Autodesk Fusion 360 part; units mm, degrees
(part 3 of 4)
  spline S333 degree 3 poles (-231.1347, 101.123) (-229.8927, 98.7978) (-228.9901, 97.7435) (-226.7371, 95.9744) knots 0 0 0 0 1 1 1 1
  spline S334 degree 3 poles (-226.7371, 95.9744) (-226.2605, 95.6061) (-225.5529, 95.0284) (-225.1629, 94.6962) knots 0 0 0 0 1 1 1 1
  spline S335 degree 3 poles (-225.1629, 94.6962) (-224.383, 94.0175) (-224.3903, 94.0319) (-224.5708, 93.2665) knots 0 0 0 0 1 1 1 1
  spline S336 degree 3 poles (-224.5708, 93.2665) (-224.8163, 92.2483) (-224.6574, 91.194) (-224.1087, 90.1614) knots 0 0 0 0 1 1 1 1
  spline S337 degree 3 poles (-224.1087, 90.1614) (-223.762, 89.5115) (-223.7548, 89.4754) (-223.7332, 88.3417) knots 0 0 0 0 1 1 1 1
  line L62 (-223.7332, 88.3417) -> (-223.7115, 87.3886)
  line L63 (-223.7115, 87.3886) -> (-224.1231, 87.1719)
  spline S338 degree 3 poles (-224.1231, 87.1719) (-224.9607, 86.7314) (-225.9717, 85.8144) (-227.0765, 84.4929) knots 0 0 0 0 1 1 1 1
  spline S339 degree 3 poles (-227.0765, 84.4929) (-227.8564, 83.5686) (-228.8168, 82.11) (-229.1128, 81.4168) knots 0 0 0 0 1 1 1 1
  spline S340 degree 3 poles (-229.1128, 81.4168) (-229.2428, 81.099) (-229.5244, 80.4708) (-229.7266, 80.0159) knots 0 0 0 0 1 1 1 1
  spline S341 degree 3 poles (-229.7266, 80.0159) (-230.6942, 77.8857) (-231.1925, 75.6399) (-231.0264, 74.1668) knots 0 0 0 0 1 1 1 1
  spline S342 degree 3 poles (-231.0264, 74.1668) (-230.817, 72.3038) (-229.9071, 71.3073) (-228.1091, 70.9679) knots 0 0 0 0 1 1 1 1
  spline S343 degree 3 poles (-228.1091, 70.9679) (-226.441, 70.6502) (-226.4844, 70.6502) (-225.7839, 70.9318) knots 0 0 0 0 1 1 1 1
  spline S344 degree 3 poles (-225.7839, 70.9318) (-225.4445, 71.069) (-225.3796, 71.0762) (-225.1196, 70.9896) knots 0 0 0 0 1 1 1 1
  spline S345 degree 3 poles (-225.1196, 70.9896) (-224.8669, 70.9101) (-224.7513, 70.9101) (-224.282, 71.0257) knots 0 0 0 0 1 1 1 1
  spline S346 degree 3 poles (-224.282, 71.0257) (-223.6754, 71.1701) (-223.1266, 71.1412) (-222.6717, 70.9463) knots 0 0 0 0 1 1 1 1
  spline S347 degree 3 poles (-222.6717, 70.9463) (-222.5272, 70.8813) (-222.1806, 70.8018) (-221.9062, 70.7657) knots 0 0 0 0 1 1 1 1
  spline S348 degree 3 poles (-221.9062, 70.7657) (-221.6174, 70.7296) (-221.1986, 70.6069) (-220.9458, 70.4913) knots 0 0 0 0 1 1 1 1
  spline S349 degree 3 poles (-220.9458, 70.4913) (-220.4692, 70.2603) (-219.7977, 69.6826) (-219.545, 69.2854) knots 0 0 0 0 1 1 1 1
  spline S350 degree 3 poles (-219.545, 69.2854) (-219.3428, 68.9532) (-219.1839, 68.9244) (-218.729, 69.1338) knots 0 0 0 0 1 1 1 1
  spline S351 degree 3 poles (-218.729, 69.1338) (-217.3498, 69.762) (-215.9489, 71.069) (-214.3964, 73.1559) knots 0 0 0 0 1 1 1 1
  spline S352 degree 3 poles (-214.3964, 73.1559) (-213.8548, 73.8924) (-213.3782, 74.499) (-213.3421, 74.5134) knots 0 0 0 0 1 1 1 1
  spline S353 degree 3 poles (-213.3421, 74.5134) (-213.2338, 74.5496) (-206.4099, 71.1268) (-206.4099, 71.0329) knots 0 0 0 0 1 1 1 1
  spline S354 degree 3 poles (-206.4099, 71.0329) (-206.4099, 70.9896) (-206.4821, 70.8379) (-206.5688, 70.7007) knots 0 0 0 0 1 1 1 1
  spline S355 degree 3 poles (-206.5688, 70.7007) (-206.9731, 70.0364) (-207.2403, 69.5165) (-207.7747, 68.3322) knots 0 0 0 0 1 1 1 1
  spline S356 degree 3 poles (-207.7747, 68.3322) (-208.4318, 66.8664) (-208.5618, 66.462) (-208.6195, 65.7543) knots 0 0 0 0 1 1 1 1
  spline S357 degree 3 poles (-208.6195, 65.7543) (-208.6484, 65.3644) (-208.6268, 65.1622) (-208.5257, 64.8878) knots 0 0 0 0 1 1 1 1
  spline S358 degree 3 poles (-208.5257, 64.8878) (-208.4101, 64.5701) (-208.3596, 64.5268) (-208.1646, 64.5051) knots 0 0 0 0 1 1 1 1
  spline S359 degree 3 poles (-208.1646, 64.5051) (-207.8324, 64.469) (-207.6591, 64.2307) (-207.5364, 63.6458) knots 0 0 0 0 1 1 1 1
  spline S360 degree 3 poles (-207.5364, 63.6458) (-207.4064, 63.0031) (-207.2692, 62.7432) (-206.9731, 62.5265) knots 0 0 0 0 1 1 1 1
  spline S361 degree 3 poles (-206.9731, 62.5265) (-206.7421, 62.3677) (-206.6843, 62.3604) (-205.3267, 62.3604) knots 0 0 0 0 1 1 1 1
  spline S362 degree 3 poles (-205.3267, 62.3604) (-203.9692, 62.3604) (-203.9114, 62.3532) (-203.6803, 62.1944) knots 0 0 0 0 1 1 1 1
  spline S363 degree 3 poles (-203.6803, 62.1944) (-203.5504, 62.1005) (-203.3626, 61.8622) (-203.2687, 61.6672) knots 0 0 0 0 1 1 1 1
  spline S364 degree 3 poles (-203.2687, 61.6672) (-203.0377, 61.2195) (-202.8716, 61.1256) (-202.5033, 61.234) knots 0 0 0 0 1 1 1 1
  spline S365 degree 3 poles (-202.5033, 61.234) (-202.0773, 61.3639) (-201.5429, 61.9055) (-200.597, 63.1764) knots 0 0 0 0 1 1 1 1
  spline S366 degree 3 poles (-200.597, 63.1764) (-199.586, 64.5268) (-198.6617, 66.0937) (-198.2862, 67.0902) knots 0 0 0 0 1 1 1 1
  spline S367 degree 3 poles (-198.2862, 67.0902) (-197.9396, 68.0001) (-197.6724, 68.8016) (-197.6724, 68.9244) knots 0 0 0 0 1 1 1 1
  spline S368 degree 3 poles (-197.6724, 68.9244) (-197.6724, 69.1627) (-197.4847, 69.1915) (-197.0587, 69.0038) knots 0 0 0 0 1 1 1 1
  spline S369 degree 3 poles (-197.0587, 69.0038) (-196.5893, 68.7944) (-194.9285, 68.3467) (-193.4409, 68.029) knots 0 0 0 0 1 1 1 1
  spline S370 degree 3 poles (-193.4409, 68.029) (-192.1772, 67.7546) (-191.8956, 67.6029) (-191.7512, 67.1263) knots 0 0 0 0 1 1 1 1
  spline S371 degree 3 poles (-191.7512, 67.1263) (-191.6718, 66.8664) (-191.5346, 66.657) (-191.2168, 66.3392) knots 0 0 0 0 1 1 1 1
  line L64 (-191.2168, 66.3392) -> (-190.7908, 65.906)
  line L65 (-190.7908, 65.906) -> (-190.2059, 65.906)
  spline S372 degree 3 poles (-190.2059, 65.906) (-189.7149, 65.8988) (-189.5849, 65.8699) (-189.3899, 65.7327) knots 0 0 0 0 1 1 1 1
  spline S373 degree 3 poles (-189.3899, 65.7327) (-188.9567, 65.4222) (-188.8267, 65.1622) (-188.8267, 64.599) knots 0 0 0 0 1 1 1 1
  line L66 (-188.8267, 64.599) -> (-188.8267, 64.0935)
  line L67 (-188.8267, 64.0935) -> (-188.4295, 64.0718)
  spline S374 degree 3 poles (-188.4295, 64.0718) (-187.7291, 64.0285) (-187.0214, 64.4473) (-186.6748, 65.0972) knots 0 0 0 0 1 1 1 1
  spline S375 degree 3 poles (-186.6748, 65.0972) (-186.4943, 65.4438) (-186.4654, 66.0648) (-186.617, 66.4259) knots 0 0 0 0 1 1 1 1
  spline S376 degree 3 poles (-186.617, 66.4259) (-186.6748, 66.5559) (-186.7037, 66.6786) (-186.682, 66.6931) knots 0 0 0 0 1 1 1 1
  spline S377 degree 3 poles (-186.682, 66.6931) (-186.6676, 66.7075) (-186.3499, 66.6786) (-185.9744, 66.6209) knots 0 0 0 0 1 1 1 1
  spline S378 degree 3 poles (-185.9744, 66.6209) (-184.0825, 66.3392) (-181.8223, 66.3104) (-181.1218, 66.5486) knots 0 0 0 0 1 1 1 1
  spline S379 degree 3 poles (-181.1218, 66.5486) (-180.8835, 66.6281) (-180.7391, 66.6353) (-180.5514, 66.5847) knots 0 0 0 0 1 1 1 1
  spline S380 degree 3 poles (-180.5514, 66.5847) (-179.8798, 66.3898) (-178.4789, 66.6281) (-178.0746, 67.0036) knots 0 0 0 0 1 1 1 1
  spline S381 degree 3 poles (-178.0746, 67.0036) (-177.959, 67.1119) (-177.8218, 67.2996) (-177.7713, 67.4296) knots 0 0 0 0 1 1 1 1
  spline S382 degree 3 poles (-177.7713, 67.4296) (-177.5546, 67.9279) (-177.7135, 69.2204) (-178.0746, 69.957) knots 0 0 0 0 1 1 1 1
  spline S383 degree 3 poles (-178.0746, 69.957) (-178.1757, 70.1664) (-178.4934, 70.5924) (-178.775, 70.9029) knots 0 0 0 0 1 1 1 1
  spline S384 degree 3 poles (-178.775, 70.9029) (-179.6632, 71.8705) (-179.7282, 72.2605) (-179.6632, 76.4776) knots 0 0 0 0 1 1 1 1
  spline S385 degree 3 poles (-179.6632, 76.4776) (-179.6343, 78.1673) (-179.5838, 80.2758) (-179.5476, 81.1712) knots 0 0 0 0 1 1 1 1
  spline S386 degree 3 poles (-179.5476, 81.1712) (-179.5115, 82.0666) (-179.4538, 83.4675) (-179.4321, 84.2907) knots 0 0 0 0 1 1 1 1
  line L68 (-179.4321, 84.2907) -> (-179.3816, 85.7783)
  line L69 (-179.3816, 85.7783) -> (-179.6054, 86.0021)
  spline S387 degree 3 poles (-179.6054, 86.0021) (-179.887, 86.2837) (-180.1759, 86.2982) (-180.4214, 86.0382) knots 0 0 0 0 1 1 1 1
  line L70 (-180.4214, 86.0382) -> (-180.5947, 85.8505)
  line L71 (-180.5947, 85.8505) -> (-180.6813, 82.6299)
  spline S388 degree 3 poles (-180.6813, 82.6299) (-180.7247, 80.8535) (-180.768, 79.0338) (-180.768, 78.5933) knots 0 0 0 0 1 1 1 1
  spline S389 degree 3 poles (-180.768, 78.5933) (-180.7752, 78.1456) (-180.8041, 77.7774) (-180.833, 77.7774) knots 0 0 0 0 1 1 1 1
  spline S390 degree 3 poles (-180.833, 77.7774) (-180.9774, 77.7774) (-181.3457, 79.6981) (-181.5334, 81.4601) knots 0 0 0 0 1 1 1 1
  spline S391 degree 3 poles (-181.5334, 81.4601) (-181.7789, 83.8069) (-182.0245, 86.7098) (-182.1111, 88.3562) knots 0 0 0 0 1 1 1 1
  spline S392 degree 3 poles (-182.1111, 88.3562) (-182.1689, 89.4104) (-182.2411, 89.7282) (-182.4866, 89.952) knots 0 0 0 0 1 1 1 1
  spline S393 degree 3 poles (-182.4866, 89.952) (-182.7177, 90.1686) (-183.086, 90.1831) (-183.2665, 89.9809) knots 0 0 0 0 1 1 1 1
  spline S394 degree 3 poles (-183.2665, 89.9809) (-183.3892, 89.8437) (-183.3892, 89.757) (-183.317, 88.6306) knots 0 0 0 0 1 1 1 1
  spline S395 degree 3 poles (-183.317, 88.6306) (-183.2665, 87.959) (-183.1798, 86.7026) (-183.1221, 85.8288) knots 0 0 0 0 1 1 1 1
  spline S396 degree 3 poles (-183.1221, 85.8288) (-183.0643, 84.9551) (-182.9993, 84.1246) (-182.9704, 83.9874) knots 0 0 0 0 1 1 1 1
  spline S397 degree 3 poles (-182.9704, 83.9874) (-182.9488, 83.8214) (-182.956, 83.7636) (-182.9993, 83.8069) knots 0 0 0 0 1 1 1 1
  spline S398 degree 3 poles (-182.9993, 83.8069) (-183.0426, 83.8502) (-183.4614, 84.7095) (-183.9308, 85.7205) knots 0 0 0 0 1 1 1 1
  spline S399 degree 3 poles (-183.9308, 85.7205) (-184.4074, 86.7314) (-185.0573, 88.0457) (-185.3822, 88.6378) knots 0 0 0 0 1 1 1 1
  spline S400 degree 3 poles (-185.3822, 88.6378) (-185.7, 89.2371) (-185.9527, 89.7498) (-185.931, 89.7787) knots 0 0 0 0 1 1 1 1
  spline S401 degree 3 poles (-185.931, 89.7787) (-185.9094, 89.8076) (-185.7938, 89.8365) (-185.6711, 89.8365) knots 0 0 0 0 1 1 1 1
  spline S402 degree 3 poles (-185.6711, 89.8365) (-185.3317, 89.8365) (-184.9779, 90.0459) (-184.4363, 90.5514) knots 0 0 0 0 1 1 1 1
  spline S403 degree 3 poles (-184.4363, 90.5514) (-182.4433, 92.4288) (-181.7212, 95.6422) (-182.8188, 97.7435) knots 0 0 0 0 1 1 1 1
  spline S404 degree 3 poles (-182.8188, 97.7435) (-183.3026, 98.675) (-184.4652, 99.5416) (-185.5194, 99.7654) knots 0 0 0 0 1 1 1 1
  spline S405 degree 3 poles (-185.5194, 99.7654) (-188.0757, 100.307) (-190.5453, 98.7906) (-191.2963, 96.2127) knots 0 0 0 0 1 1 1 1
  spline S406 degree 3 poles (-191.2963, 96.2127) (-191.3685, 95.9599) (-191.4407, 95.7577) (-191.4624, 95.7577) knots 0 0 0 0 1 1 1 1
  spline S407 degree 3 poles (-191.4624, 95.7577) (-191.484, 95.7577) (-191.7584, 95.9744) (-192.0761, 96.2415) knots 0 0 0 0 1 1 1 1
  spline S408 degree 3 poles (-192.0761, 96.2415) (-193.477, 97.4113) (-194.8274, 98.3212) (-196.0983, 98.935) knots 0 0 0 0 1 1 1 1
  spline S409 degree 3 poles (-196.0983, 98.935) (-196.5965, 99.1805) (-196.777, 99.3033) (-196.712, 99.3538) knots 0 0 0 0 1 1 1 1
  spline S410 degree 3 poles (-196.712, 99.3538) (-196.6615, 99.3899) (-196.3943, 99.5416) (-196.1127, 99.6788) knots 0 0 0 0 1 1 1 1
  spline S411 degree 3 poles (-196.1127, 99.6788) (-195.0873, 100.1987) (-194.3291, 101.3179) (-194.0908, 102.6899) knots 0 0 0 0 1 1 1 1
  spline S412 degree 3 poles (-194.0908, 102.6899) (-193.9536, 103.4987) (-193.9897, 104.7263) (-194.1702, 105.3978) knots 0 0 0 0 1 1 1 1
  spline S413 degree 3 poles (-194.1702, 105.3978) (-194.4446, 106.4376) (-195.0873, 107.4702) (-196.026, 108.409) knots 0 0 0 0 1 1 1 1
  spline S414 degree 3 poles (-196.026, 108.409) (-196.9937, 109.3622) (-197.8891, 109.6943) (-199.5355, 109.6943) knots 0 0 0 0 1 1 1 1
  line L72 (-199.5355, 109.6943) -> (-200.4237, 109.6943)
  line L73 (-200.4237, 109.6943) -> (-201.1313, 110.3659)
  spline S415 degree 3 poles (-201.1313, 110.3659) (-202.5394, 111.6873) (-203.7526, 112.1423) (-205.3556, 111.9473) knots 0 0 0 0 1 1 1 1
  spline S416 degree 3 poles (-205.3556, 111.9473) (-206.6337, 111.7884) (-207.5003, 111.3913) (-208.2946, 110.6114) knots 0 0 0 0 1 1 1 1
  spline S417 degree 3 poles (-208.2946, 110.6114) (-208.9806, 109.9254) (-209.4788, 108.7123) (-209.6521, 107.2681) knots 0 0 0 0 1 1 1 1
  spline S418 degree 3 poles (-209.6521, 107.2681) (-209.7749, 106.2427) (-209.5944, 105.0368) (-209.1756, 104.1341) knots 0 0 0 0 1 1 1 1
  spline S419 degree 3 poles (-209.1756, 104.1341) (-208.9517, 103.6575) (-208.0274, 102.7188) (-207.3703, 102.2928) knots 0 0 0 0 1 1 1 1
  spline S420 degree 3 poles (-207.3703, 102.2928) (-207.1176, 102.1339) (-206.9154, 101.9823) (-206.9154, 101.9606) knots 0 0 0 0 1 1 1 1
  spline S421 degree 3 poles (-206.9154, 101.9606) (-206.9154, 101.9317) (-207.7169, 101.8956) (-208.699, 101.8739) knots 0 0 0 0 1 1 1 1
  spline S422 degree 3 poles (-208.699, 101.8739) (-210.7786, 101.8306) (-211.2697, 101.7512) (-213.0171, 101.1591) knots 0 0 0 0 1 1 1 1
  spline S423 degree 3 poles (-213.0171, 101.1591) (-214.6419, 100.6103) (-215.8333, 100.0903) (-217.0104, 99.4332) knots 0 0 0 0 1 1 1 1
  spline S424 degree 3 poles (-217.0104, 99.4332) (-218.4113, 98.6534) (-219.2561, 98.0685) (-219.8121, 97.5052) knots 0 0 0 0 1 1 1 1
  spline S425 degree 3 poles (-219.8121, 97.5052) (-220.2598, 97.0503) (-220.2815, 97.0431) (-220.4909, 97.1297) knots 0 0 0 0 1 1 1 1
  spline S426 degree 3 poles (-220.4909, 97.1297) (-220.8159, 97.2669) (-221.473, 97.1875) (-221.9857, 96.9564) knots 0 0 0 0 1 1 1 1
  line L74 (-221.9857, 96.9564) -> (-222.4334, 96.7542)
  line L75 (-222.4334, 96.7542) -> (-222.8161, 96.9564)
  spline S427 degree 3 poles (-222.8161, 96.9564) (-223.0833, 97.1008) (-223.6537, 97.6135) (-224.7152, 98.6822) knots 0 0 0 0 1 1 1 1
  spline S428 degree 3 poles (-224.7152, 98.6822) (-226.2605, 100.2275) (-226.8021, 100.8919) (-227.3292, 101.8956) knots 0 0 0 0 1 1 1 1
  spline S429 degree 3 poles (-227.3292, 101.8956) (-227.4881, 102.1917) (-227.7481, 102.6827) (-227.9141, 102.9788) knots 0 0 0 0 1 1 1 1
  spline S430 degree 3 poles (-227.9141, 102.9788) (-228.073, 103.2748) (-228.3979, 103.9897) (-228.6362, 104.5674) knots 0 0 0 0 1 1 1 1
  spline S431 degree 3 poles (-228.6362, 104.5674) (-229.4522, 106.5315) (-230.0082, 107.7808) (-230.8025, 109.4055) knots 0 0 0 0 1 1 1 1
  spline S432 degree 3 poles (-230.8025, 109.4055) (-231.2358, 110.3009) (-231.7918, 111.4924) (-232.0373, 112.0628) knots 0 0 0 0 1 1 1 1
  spline S433 degree 3 poles (-232.0373, 112.0628) (-233.2216, 114.814) (-234.3914, 116.9298) (-235.7129, 118.6845) knots 0 0 0 0 1 1 1 1
  spline S434 degree 3 poles (-235.7129, 118.6845) (-236.3411, 119.5222) (-238.4568, 121.6957) (-239.3017, 122.3817) knots 0 0 0 0 1 1 1 1
  spline S435 degree 3 poles (-239.3017, 122.3817) (-240.0527, 122.9883) (-242.0313, 123.9342) (-243.0566, 124.1725) knots 0 0 0 0 1 1 1 1
  spline S436 degree 3 poles (-243.0566, 124.1725) (-243.5982, 124.3025) (-244.3998, 124.3025) (-244.8258, 124.1725) knots 0 0 0 0 1 1 1 1
  spline S437 degree 3 poles (-242.6956, 122.8511) (-242.0457, 122.62) (-241.7857, 122.49) (-241.042, 122.0062) knots 0 0 0 0 1 1 1 1
  line L76 (-241.042, 122.0062) -> (-240.4282, 121.6018)
  line L77 (-240.4282, 121.6018) -> (-240.6015, 121.3419)
  spline S438 degree 3 poles (-240.6015, 121.3419) (-240.7026, 121.2047) (-240.8542, 120.8942) (-240.9337, 120.6631) knots 0 0 0 0 1 1 1 1
  spline S439 degree 3 poles (-240.9337, 120.6631) (-241.0203, 120.4248) (-241.107, 120.237) (-241.1286, 120.237) knots 0 0 0 0 1 1 1 1
  spline S440 degree 3 poles (-241.1286, 120.237) (-241.1503, 120.237) (-241.4102, 120.3959) (-241.7135, 120.5836) knots 0 0 0 0 1 1 1 1
  spline S441 degree 3 poles (-241.7135, 120.5836) (-242.0168, 120.7786) (-242.5512, 121.0963) (-242.905, 121.2913) knots 0 0 0 0 1 1 1 1
  spline S442 degree 3 poles (-242.905, 121.2913) (-243.6415, 121.6957) (-244.1903, 122.1578) (-244.3203, 122.4756) knots 0 0 0 0 1 1 1 1
  spline S443 degree 3 poles (-244.3203, 122.4756) (-244.3998, 122.6705) (-244.3925, 122.7139) (-244.2842, 122.8366) knots 0 0 0 0 1 1 1 1
  spline S444 degree 3 poles (-244.2842, 122.8366) (-243.9954, 123.1543) (-243.5621, 123.1616) (-242.6956, 122.8511) knots 0 0 0 0 1 1 1 1
  spline S445 degree 3 poles (-238.2691, 119.811) (-237.5903, 119.1394) (-237.0271, 118.5618) (-237.0271, 118.5184) knots 0 0 0 0 1 1 1 1
  spline S446 degree 3 poles (-237.0271, 118.5184) (-237.0271, 118.4823) (-237.0993, 118.4029) (-237.1859, 118.3379) knots 0 0 0 0 1 1 1 1
  spline S447 degree 3 poles (-237.1859, 118.3379) (-237.2798, 118.2801) (-237.547, 118.0491) (-237.7853, 117.818) knots 0 0 0 0 1 1 1 1
  line L78 (-237.7853, 117.818) -> (-238.2113, 117.4064)
  line L79 (-238.2113, 117.4064) -> (-238.6085, 117.8613)
  spline S448 degree 3 poles (-238.6085, 117.8613) (-238.8251, 118.1141) (-239.28, 118.5906) (-239.6194, 118.9156) knots 0 0 0 0 1 1 1 1
  line L80 (-239.6194, 118.9156) -> (-240.2404, 119.5005)
  line L81 (-240.2404, 119.5005) -> (-240.1032, 119.9049)
  spline S449 degree 3 poles (-240.1032, 119.9049) (-239.9877, 120.2443) (-239.5905, 121.0313) (-239.5328, 121.0313) knots 0 0 0 0 1 1 1 1
  spline S450 degree 3 poles (-239.5328, 121.0313) (-239.5256, 121.0313) (-238.9551, 120.4826) (-238.2691, 119.811) knots 0 0 0 0 1 1 1 1
  spline S451 degree 3 poles (-235.8862, 116.937) (-235.3157, 116.0922) (-234.2831, 114.2075) (-234.2831, 114.0125) knots 0 0 0 0 1 1 1 1
  spline S452 degree 3 poles (-234.2831, 114.0125) (-234.2831, 113.962) (-234.4347, 113.7237) (-234.6225, 113.4926) knots 0 0 0 0 1 1 1 1
  line L82 (-234.6225, 113.4926) -> (-234.9546, 113.0593)
  line L83 (-234.9546, 113.0593) -> (-235.2435, 113.3843)
  spline S453 degree 3 poles (-235.2435, 113.3843) (-235.4023, 113.5576) (-235.8356, 114.1569) (-236.2039, 114.7129) knots 0 0 0 0 1 1 1 1
  spline S454 degree 3 poles (-236.2039, 114.7129) (-236.5794, 115.269) (-236.9838, 115.8611) (-237.1065, 116.0272) knots 0 0 0 0 1 1 1 1
  spline S455 degree 3 poles (-237.1065, 116.0272) (-237.3159, 116.3016) (-237.3231, 116.3449) (-237.2509, 116.576) knots 0 0 0 0 1 1 1 1
  spline S456 degree 3 poles (-237.2509, 116.576) (-237.1571, 116.8431) (-236.9621, 117.0526) (-236.6299, 117.2259) knots 0 0 0 0 1 1 1 1
  spline S457 degree 3 poles (-236.6299, 117.2259) (-236.2761, 117.4136) (-236.1822, 117.3775) (-235.8862, 116.937) knots 0 0 0 0 1 1 1 1
  spline S458 degree 3 poles (-232.8533, 111.1674) (-232.4489, 110.2503) (-232.1023, 109.4488) (-232.0807, 109.391) knots 0 0 0 0 1 1 1 1
  spline S459 degree 3 poles (-232.0807, 109.391) (-232.0229, 109.2394) (-232.5428, 109.0011) (-232.6656, 109.1311) knots 0 0 0 0 1 1 1 1
  spline S460 degree 3 poles (-232.6656, 109.1311) (-232.7161, 109.1816) (-232.9616, 109.6871) (-233.2216, 110.2503) knots 0 0 0 0 1 1 1 1
  spline S461 degree 3 poles (-233.2216, 110.2503) (-233.4743, 110.8064) (-233.8209, 111.4707) (-233.987, 111.7162) knots 0 0 0 0 1 1 1 1
  spline S462 degree 3 poles (-233.987, 111.7162) (-234.182, 111.9978) (-234.2759, 112.2072) (-234.247, 112.2867) knots 0 0 0 0 1 1 1 1
  spline S463 degree 3 poles (-234.247, 112.2867) (-234.1892, 112.4672) (-233.691, 112.9582) (-233.6332, 112.8932) knots 0 0 0 0 1 1 1 1
  spline S464 degree 3 poles (-233.6332, 112.8932) (-233.6043, 112.8571) (-233.2577, 112.0845) (-232.8533, 111.1674) knots 0 0 0 0 1 1 1 1
  spline S465 degree 3 poles (-203.897, 110.1709) (-202.9366, 109.8243) (-202.2361, 109.2394) (-201.8173, 108.4379) knots 0 0 0 0 1 1 1 1
  spline S466 degree 3 poles (-201.8173, 108.4379) (-201.6801, 108.1707) (-201.5646, 108.0335) (-201.4707, 108.0335) knots 0 0 0 0 1 1 1 1
  spline S467 degree 3 poles (-201.4707, 108.0335) (-201.3985, 108.0335) (-200.9364, 108.084) (-200.4453, 108.1562) knots 0 0 0 0 1 1 1 1
  spline S468 degree 3 poles (-200.4453, 108.1562) (-199.3477, 108.3007) (-198.7339, 108.2357) (-198.0046, 107.8963) knots 0 0 0 0 1 1 1 1
  spline S469 degree 3 poles (-198.0046, 107.8963) (-197.2825, 107.5641) (-196.4449, 106.7193) (-196.026, 105.9033) knots 0 0 0 0 1 1 1 1
  spline S470 degree 3 poles (-196.026, 105.9033) (-195.6794, 105.2173) (-195.5422, 104.5746) (-195.5495, 103.6648) knots 0 0 0 0 1 1 1 1
  spline S471 degree 3 poles (-195.5495, 103.6648) (-195.5567, 102.9354) (-195.5783, 102.726) (-195.7228, 102.365) knots 0 0 0 0 1 1 1 1
  spline S472 degree 3 poles (-195.7228, 102.365) (-195.9538, 101.7656) (-196.611, 101.1157) (-197.2031, 100.8919) knots 0 0 0 0 1 1 1 1
  spline S473 degree 3 poles (-197.2031, 100.8919) (-198.0696, 100.5669) (-199.3116, 100.8197) (-200.4092, 101.549) knots 0 0 0 0 1 1 1 1
  line L84 (-200.4092, 101.549) -> (-200.8786, 101.8595)
  line L85 (-200.8786, 101.8595) -> (-200.8569, 102.4372)
  spline S474 degree 3 poles (-200.8569, 102.4372) (-200.8425, 103.1376) (-200.9869, 103.6648) (-201.2613, 103.9319) knots 0 0 0 0 1 1 1 1
  spline S475 degree 3 poles (-201.2613, 103.9319) (-201.7451, 104.3941) (-202.8644, 104.7046) (-203.5287, 104.5602) knots 0 0 0 0 1 1 1 1
  spline S476 degree 3 poles (-203.5287, 104.5602) (-203.7959, 104.5024) (-203.9836, 104.3941) (-204.2652, 104.1341) knots 0 0 0 0 1 1 1 1
  line L86 (-204.2652, 104.1341) -> (-204.6407, 103.7947)
  line L87 (-204.6407, 103.7947) -> (-204.814, 104.0691)
  spline S477 degree 3 poles (-204.814, 104.0691) (-204.9151, 104.2208) (-205.009, 104.3291) (-205.0379, 104.3147) knots 0 0 0 0 1 1 1 1
  spline S478 degree 3 poles (-205.0379, 104.3147) (-205.0668, 104.3002) (-205.0884, 104.3291) (-205.0884, 104.3796) knots 0 0 0 0 1 1 1 1
  spline S479 degree 3 poles (-205.0884, 104.3796) (-205.0884, 104.4446) (-204.9657, 104.5024) (-204.7924, 104.5241) knots 0 0 0 0 1 1 1 1
  spline S480 degree 3 poles (-204.7924, 104.5241) (-204.1425, 104.6324) (-203.4926, 105.0729) (-203.2254, 105.5856) knots 0 0 0 0 1 1 1 1
  spline S481 degree 3 poles (-203.2254, 105.5856) (-203.0377, 105.9611) (-203.0377, 106.6759) (-203.2399, 107.2031) knots 0 0 0 0 1 1 1 1
  spline S482 degree 3 poles (-203.2399, 107.2031) (-203.3337, 107.4558) (-203.5143, 107.7374) (-203.7381, 107.9613) knots 0 0 0 0 1 1 1 1
  spline S483 degree 3 poles (-203.7381, 107.9613) (-204.5469, 108.7917) (-205.6084, 108.9217) (-206.4316, 108.2934) knots 0 0 0 0 1 1 1 1
  spline S484 degree 3 poles (-206.4316, 108.2934) (-206.7565, 108.0479) (-206.8576, 108.1346) (-206.8865, 108.6762) knots 0 0 0 0 1 1 1 1
  spline S485 degree 3 poles (-206.8865, 108.6762) (-206.9009, 108.9289) (-206.8793, 109.1166) (-206.8432, 109.1166) knots 0 0 0 0 1 1 1 1
  spline S486 degree 3 poles (-206.8432, 109.1166) (-206.7998, 109.1166) (-206.7782, 109.1383) (-206.7854, 109.1744) knots 0 0 0 0 1 1 1 1
  spline S487 degree 3 poles (-206.7854, 109.1744) (-206.8071, 109.2683) (-206.6121, 109.8749) (-206.5327, 109.9759) knots 0 0 0 0 1 1 1 1
  spline S488 degree 3 poles (-206.5327, 109.9759) (-206.4821, 110.0337) (-206.316, 110.142) (-206.1572, 110.2142) knots 0 0 0 0 1 1 1 1
  spline S489 degree 3 poles (-206.1572, 110.2142) (-205.9116, 110.3298) (-205.7456, 110.3442) (-205.0379, 110.3153) knots 0 0 0 0 1 1 1 1
  spline S490 degree 3 poles (-205.0379, 110.3153) (-204.5396, 110.3009) (-204.0847, 110.2431) (-203.897, 110.1709) knots 0 0 0 0 1 1 1 1
  spline S491 degree 3 poles (-231.4741, 108.2718) (-231.3225, 108.1418) (-230.1093, 105.2967) (-230.0371, 104.8996) knots 0 0 0 0 1 1 1 1
  spline S492 degree 3 poles (-230.0371, 104.8996) (-230.0155, 104.7479) (-230.0371, 104.6613) (-230.1382, 104.5891) knots 0 0 0 0 1 1 1 1
  spline S493 degree 3 poles (-230.1382, 104.5891) (-230.391, 104.4013) (-230.4993, 104.4735) (-230.7448, 105.0223) knots 0 0 0 0 1 1 1 1
  spline S494 degree 3 poles (-230.7448, 105.0223) (-231.0914, 105.8022) (-231.1419, 105.9177) (-231.4308, 106.6254) knots 0 0 0 0 1 1 1 1
  spline S495 degree 3 poles (-231.4308, 106.6254) (-231.5824, 106.9864) (-231.7918, 107.4702) (-231.9074, 107.7085) knots 0 0 0 0 1 1 1 1
  line L88 (-231.9074, 107.7085) -> (-232.1096, 108.1418)
  line L89 (-232.1096, 108.1418) -> (-231.9579, 108.2718)
  spline S496 degree 3 poles (-231.9579, 108.2718) (-231.8785, 108.3368) (-231.7702, 108.3945) (-231.7196, 108.3945) knots 0 0 0 0 1 1 1 1
  spline S497 degree 3 poles (-231.7196, 108.3945) (-231.6691, 108.3945) (-231.5608, 108.3368) (-231.4741, 108.2718) knots 0 0 0 0 1 1 1 1
  spline S498 degree 3 poles (-204.6552, 107.167) (-204.3302, 106.9142) (-204.3086, 106.3077) (-204.6046, 106.0116) knots 0 0 0 0 1 1 1 1
  spline S499 degree 3 poles (-204.6046, 106.0116) (-204.879, 105.7372) (-205.5361, 105.8672) (-205.7311, 106.2355) knots 0 0 0 0 1 1 1 1
  spline S500 degree 3 poles (-205.7311, 106.2355) (-205.9405, 106.647) (-205.825, 107.0442) (-205.4495, 107.2031) knots 0 0 0 0 1 1 1 1
  spline S501 degree 3 poles (-205.4495, 107.2031) (-205.1246, 107.3475) (-204.8718, 107.333) (-204.6552, 107.167) knots 0 0 0 0 1 1 1 1
  spline S502 degree 3 poles (-207.8758, 105.7083) (-207.8974, 105.6505) (-207.9191, 105.6722) (-207.9191, 105.7516) knots 0 0 0 0 1 1 1 1
  spline S503 degree 3 poles (-207.9191, 105.7516) (-207.9263, 105.8311) (-207.9046, 105.8744) (-207.883, 105.8455) knots 0 0 0 0 1 1 1 1
  spline S504 degree 3 poles (-207.883, 105.8455) (-207.8613, 105.8239) (-207.8541, 105.7589) (-207.8758, 105.7083) knots 0 0 0 0 1 1 1 1
  spline S505 degree 3 poles (-207.5075, 104.8201) (-207.5292, 104.7985) (-207.5725, 104.8346) (-207.5941, 104.9068) knots 0 0 0 0 1 1 1 1
  spline S506 degree 3 poles (-207.5941, 104.9068) (-207.6375, 105.0079) (-207.6302, 105.0151) (-207.558, 104.9501) knots 0 0 0 0 1 1 1 1
  spline S507 degree 3 poles (-207.558, 104.9501) (-207.5075, 104.8996) (-207.4858, 104.8418) (-207.5075, 104.8201) knots 0 0 0 0 1 1 1 1
  spline S508 degree 3 poles (-228.9323, 102.5383) (-228.6146, 101.8956) (-228.1885, 101.1085) (-227.9936, 100.798) knots 0 0 0 0 1 1 1 1
  spline S509 degree 3 poles (-227.9936, 100.798) (-227.7986, 100.4803) (-227.6397, 100.177) (-227.6397, 100.1192) knots 0 0 0 0 1 1 1 1
  spline S510 degree 3 poles (-227.6397, 100.1192) (-227.6397, 99.8304) (-228.0658, 99.9676) (-228.499, 100.3936) knots 0 0 0 0 1 1 1 1
  spline S511 degree 3 poles (-228.499, 100.3936) (-228.8673, 100.7547) (-229.185, 101.289) (-229.5966, 102.235) knots 0 0 0 0 1 1 1 1
  spline S512 degree 3 poles (-229.5966, 102.235) (-229.7988, 102.7044) (-229.9938, 103.116) (-230.0299, 103.1593) knots 0 0 0 0 1 1 1 1
  spline S513 degree 3 poles (-230.0299, 103.1593) (-230.1382, 103.2676) (-230.1021, 103.3976) (-229.936, 103.5564) knots 0 0 0 0 1 1 1 1
  spline S514 degree 3 poles (-229.936, 103.5564) (-229.6255, 103.8453) (-229.5533, 103.7731) (-228.9323, 102.5383) knots 0 0 0 0 1 1 1 1
  spline S515 degree 3 poles (-205.1607, 103.1448) (-205.2112, 103.1304) (-205.2979, 103.1304) (-205.3412, 103.1448) knots 0 0 0 0 1 1 1 1
  spline S516 degree 3 poles (-205.3412, 103.1448) (-205.3917, 103.1665) (-205.3556, 103.181) (-205.2545, 103.181) knots 0 0 0 0 1 1 1 1
  spline S517 degree 3 poles (-205.2545, 103.181) (-205.1534, 103.181) (-205.1173, 103.1665) (-205.1607, 103.1448) knots 0 0 0 0 1 1 1 1
  spline S518 degree 3 poles (-202.6044, 102.6394) (-202.5178, 102.4227) (-202.5033, 102.1989) (-202.5322, 101.5707) knots 0 0 0 0 1 1 1 1
  spline S519 degree 3 poles (-202.5322, 101.5707) (-202.5539, 101.1374) (-202.6044, 100.5958) (-202.6477, 100.3792) knots 0 0 0 0 1 1 1 1
  spline S520 degree 3 poles (-202.6477, 100.3792) (-202.6838, 100.1626) (-202.7705, 99.6932) (-202.8355, 99.3394) knots 0 0 0 0 1 1 1 1
  spline S521 degree 3 poles (-202.8355, 99.3394) (-202.9799, 98.5595) (-203.2687, 97.7291) (-203.4709, 97.5124) knots 0 0 0 0 1 1 1 1
  spline S522 degree 3 poles (-203.4709, 97.5124) (-203.6442, 97.3247) (-203.9186, 97.303) (-204.3519, 97.4619) knots 0 0 0 0 1 1 1 1
  spline S523 degree 3 poles (-204.3519, 97.4619) (-204.5108, 97.5124) (-204.5685, 97.5485) (-204.4747, 97.5341) knots 0 0 0 0 1 1 1 1
  spline S524 degree 2 poles (-204.4747, 97.5341) (-204.388, 97.5197) (-204.3158, 97.5124) knots 0 0 0 1 1 1
  spline S525 degree 3 poles (-204.3158, 97.5124) (-204.3158, 97.5269) (-204.5758, 98.2273) (-204.6552, 98.4295) knots 0 0 0 0 1 1 1 1
  spline S526 degree 3 poles (-204.6552, 98.4295) (-204.6768, 98.4873) (-204.7057, 98.8267) (-204.7202, 99.1733) knots 0 0 0 0 1 1 1 1
  spline S527 degree 3 poles (-204.7202, 99.1733) (-204.7491, 99.7582) (-204.7274, 99.8593) (-204.4891, 100.5092) knots 0 0 0 0 1 1 1 1
  spline S528 degree 3 poles (-204.4891, 100.5092) (-204.1569, 101.3974) (-203.572, 102.5672) (-203.3626, 102.7549) knots 0 0 0 0 1 1 1 1
  spline S529 degree 3 poles (-203.3626, 102.7549) (-203.2687, 102.8488) (-203.1099, 102.9066) (-202.9655, 102.9066) knots 0 0 0 0 1 1 1 1
  spline S530 degree 3 poles (-202.9655, 102.9066) (-202.7488, 102.9066) (-202.7055, 102.8704) (-202.6044, 102.6394) knots 0 0 0 0 1 1 1 1
  spline S531 degree 3 poles (-204.7707, 98.8844) (-204.7924, 98.8122) (-204.8068, 98.8556) (-204.8068, 98.9711) knots 0 0 0 0 1 1 1 1
  spline S532 degree 3 poles (-204.8068, 98.9711) (-204.8068, 99.0938) (-204.7924, 99.1444) (-204.7707, 99.1011) knots 0 0 0 0 1 1 1 1
  spline S533 degree 3 poles (-204.7707, 99.1011) (-204.7563, 99.0505) (-204.7563, 98.9494) (-204.7707, 98.8844) knots 0 0 0 0 1 1 1 1
  spline S534 degree 3 poles (-183.9886, 96.5304) (-183.6781, 96.2271) (-183.4831, 95.765) (-183.5337, 95.4617) knots 0 0 0 0 1 1 1 1
  spline S535 degree 3 poles (-183.5337, 95.4617) (-183.5481, 95.3461) (-183.6853, 95.4689) (-184.1402, 95.9888) knots 0 0 0 0 1 1 1 1
  spline S536 degree 3 poles (-184.1402, 95.9888) (-184.8984, 96.8625) (-184.884, 96.8409) (-184.559, 96.8409) knots 0 0 0 0 1 1 1 1
  spline S537 degree 3 poles (-184.559, 96.8409) (-184.3424, 96.8409) (-184.2413, 96.7831) (-183.9886, 96.5304) knots 0 0 0 0 1 1 1 1
  spline S538 degree 3 poles (-184.3352, 94.6312) (-184.068, 94.3352) (-183.8369, 94.0608) (-183.8225, 94.0247) knots 0 0 0 0 1 1 1 1
  spline S539 degree 3 poles (-183.8225, 94.0247) (-183.7864, 93.9308) (-183.9525, 93.3748) (-184.0102, 93.3748) knots 0 0 0 0 1 1 1 1
  spline S540 degree 3 poles (-184.0102, 93.3748) (-184.0608, 93.3748) (-184.8984, 94.4507) (-185.0573, 94.7179) knots 0 0 0 0 1 1 1 1
  spline S541 degree 3 poles (-185.0573, 94.7179) (-185.1151, 94.8262) (-184.9995, 95.18) (-184.8984, 95.18) knots 0 0 0 0 1 1 1 1
  spline S542 degree 3 poles (-184.8984, 95.18) (-184.8623, 95.18) (-184.6096, 94.9345) (-184.3352, 94.6312) knots 0 0 0 0 1 1 1 1
  spline S543 degree 3 poles (-185.1801, 93.1293) (-184.884, 92.7321) (-184.6746, 92.3711) (-184.6746, 92.2772) knots 0 0 0 0 1 1 1 1
  spline S544 degree 3 poles (-184.6746, 92.2772) (-184.6746, 92.1255) (-185.0067, 91.7139) (-185.1223, 91.7139) knots 0 0 0 0 1 1 1 1
  spline S545 degree 3 poles (-185.1223, 91.7139) (-185.1512, 91.7139) (-185.2884, 91.9089) (-185.4328, 92.1472) knots 0 0 0 0 1 1 1 1
  spline S546 degree 3 poles (-185.4328, 92.1472) (-185.5772, 92.3855) (-185.8227, 92.7393) (-185.9816, 92.9415) knots 0 0 0 0 1 1 1 1
  spline S547 degree 3 poles (-185.9816, 92.9415) (-186.1332, 93.1365) (-186.2632, 93.3242) (-186.2632, 93.3531) knots 0 0 0 0 1 1 1 1
  spline S548 degree 3 poles (-186.2632, 93.3531) (-186.2632, 93.447) (-185.8805, 93.808) (-185.7794, 93.808) knots 0 0 0 0 1 1 1 1
  spline S549 degree 3 poles (-185.7794, 93.808) (-185.7289, 93.808) (-185.4545, 93.5048) (-185.1801, 93.1293) knots 0 0 0 0 1 1 1 1
  spline S550 degree 3 poles (-201.8823, 93.1148) (-201.904, 93.0932) (-201.969, 93.0859) (-202.0195, 93.1076) knots 0 0 0 0 1 1 1 1
  spline S551 degree 3 poles (-202.0195, 93.1076) (-202.0773, 93.1293) (-202.0556, 93.1509) (-201.9762, 93.1509) knots 0 0 0 0 1 1 1 1
  spline S552 degree 3 poles (-201.9762, 93.1509) (-201.8967, 93.1582) (-201.8534, 93.1365) (-201.8823, 93.1148) knots 0 0 0 0 1 1 1 1
  line L90 (-186.7831, 91.8945) -> (-186.061, 90.9196)
  line L91 (-186.061, 90.9196) -> (-186.2993, 90.8763)
  spline S553 degree 3 poles (-186.2993, 90.8763) (-186.4293, 90.8546) (-186.6026, 90.8546) (-186.6893, 90.8835) knots 0 0 0 0 1 1 1 1
  spline S554 degree 3 poles (-186.6893, 90.8835) (-186.8481, 90.9341) (-188.2851, 92.566) (-188.2851, 92.7032) knots 0 0 0 0 1 1 1 1
  spline S555 degree 3 poles (-188.2851, 92.7032) (-188.2851, 92.7827) (-188.1046, 92.826) (-187.6641, 92.8549) knots 0 0 0 0 1 1 1 1
  spline S556 degree 3 poles (-187.6641, 92.8549) (-187.5413, 92.8693) (-187.3464, 92.6455) (-186.7831, 91.8945) knots 0 0 0 0 1 1 1 1
  spline S557 degree 3 poles (-205.009, 92.075) (-204.9874, 91.9595) (-204.944, 91.7501) (-204.9151, 91.6273) knots 0 0 0 0 1 1 1 1
  spline S558 degree 3 poles (-204.9151, 91.6273) (-204.8863, 91.4973) (-204.879, 91.3096) (-204.8863, 91.2085) knots 0 0 0 0 1 1 1 1
  spline S559 degree 3 poles (-204.8863, 91.2085) (-204.9151, 90.9269) (-205.2762, 90.0531) (-205.5795, 89.5115) knots 0 0 0 0 1 1 1 1
  spline S560 degree 3 poles (-205.5795, 89.5115) (-205.9333, 88.8689) (-206.0055, 88.9772) (-205.9622, 90.1181) knots 0 0 0 0 1 1 1 1
  spline S561 degree 3 poles (-205.9622, 90.1181) (-205.9405, 90.8402) (-205.9044, 91.0135) (-205.7383, 91.389) knots 0 0 0 0 1 1 1 1
  spline S562 degree 3 poles (-205.7383, 91.389) (-205.5289, 91.8439) (-205.2184, 92.2916) (-205.1101, 92.2916) knots 0 0 0 0 1 1 1 1
  spline S563 degree 3 poles (-205.1101, 92.2916) (-205.0812, 92.2916) (-205.0307, 92.1978) (-205.009, 92.075) knots 0 0 0 0 1 1 1 1
  spline S564 degree 3 poles (-204.5252, 91.9089) (-204.5974, 91.8439) (-204.6046, 91.8511) (-204.5613, 91.9522) knots 0 0 0 0 1 1 1 1
  spline S565 degree 3 poles (-204.5613, 91.9522) (-204.5396, 92.0245) (-204.4963, 92.0606) (-204.4747, 92.0389) knots 0 0 0 0 1 1 1 1
  spline S566 degree 3 poles (-204.4747, 92.0389) (-204.453, 92.0172) (-204.4747, 91.9595) (-204.5252, 91.9089) knots 0 0 0 0 1 1 1 1
  spline S567 degree 3 poles (-204.0919, 89.887) (-204.1642, 89.822) (-204.1714, 89.8293) (-204.128, 89.9304) knots 0 0 0 0 1 1 1 1
  spline S568 degree 3 poles (-204.128, 89.9304) (-204.1064, 90.0026) (-204.0631, 90.0387) (-204.0414, 90.017) knots 0 0 0 0 1 1 1 1
  spline S569 degree 3 poles (-204.0414, 90.017) (-204.0197, 89.9953) (-204.0414, 89.9376) (-204.0919, 89.887) knots 0 0 0 0 1 1 1 1
  spline S570 degree 3 poles (-203.9259, 89.1938) (-203.9403, 89.1721) (-203.8825, 89.0855) (-203.7959, 88.9916) knots 0 0 0 0 1 1 1 1
  line L92 (-203.7959, 88.9916) -> (-203.637, 88.8255)
  line L93 (-203.637, 88.8255) -> (-204.1064, 87.6557)
  spline S571 degree 3 poles (-204.1064, 87.6557) (-204.3663, 87.0131) (-204.6119, 86.4787) (-204.6552, 86.4643) knots 0 0 0 0 1 1 1 1
  spline S572 degree 3 poles (-204.6552, 86.4643) (-204.7779, 86.4209) (-205.0307, 86.8975) (-205.0812, 87.2514) knots 0 0 0 0 1 1 1 1
  spline S573 degree 3 poles (-205.0812, 87.2514) (-205.139, 87.6702) (-204.9657, 88.3417) (-204.5974, 89.1144) knots 0 0 0 0 1 1 1 1
  line L94 (-204.5974, 89.1144) -> (-204.3086, 89.7282)
  line L95 (-204.3086, 89.7282) -> (-204.0992, 89.4754)
  spline S574 degree 3 poles (-204.0992, 89.4754) (-203.9836, 89.3382) (-203.9042, 89.2083) (-203.9259, 89.1938) knots 0 0 0 0 1 1 1 1
  spline S575 degree 3 poles (-200.7703, 89.4538) (-200.8425, 89.3888) (-200.8497, 89.396) (-200.8064, 89.4971) knots 0 0 0 0 1 1 1 1
  spline S576 degree 3 poles (-200.8064, 89.4971) (-200.7847, 89.5693) (-200.7414, 89.6054) (-200.7197, 89.5837) knots 0 0 0 0 1 1 1 1
  spline S577 degree 3 poles (-200.7197, 89.5837) (-200.6981, 89.5621) (-200.7197, 89.5043) (-200.7703, 89.4538) knots 0 0 0 0 1 1 1 1
  spline S578 degree 3 poles (-203.4276, 89.2949) (-203.4493, 89.2299) (-203.4854, 89.1938) (-203.4998, 89.2155) knots 0 0 0 0 1 1 1 1
  spline S579 degree 3 poles (-203.4998, 89.2155) (-203.5215, 89.2371) (-203.5143, 89.2805) (-203.4854, 89.3238) knots 0 0 0 0 1 1 1 1
  spline S580 degree 3 poles (-203.4854, 89.3238) (-203.4204, 89.4393) (-203.3771, 89.4177) (-203.4276, 89.2949) knots 0 0 0 0 1 1 1 1
  spline S581 degree 3 poles (-195.6867, 88.0096) (-195.6867, 86.717) (-196.1199, 85.6772) (-196.8565, 85.215) knots 0 0 0 0 1 1 1 1
  spline S582 degree 3 poles (-196.8565, 85.215) (-197.1525, 85.0273) (-197.6002, 84.919) (-197.6002, 85.0417) knots 0 0 0 0 1 1 1 1
  spline S583 degree 3 poles (-197.6002, 85.0417) (-197.6002, 85.0634) (-197.463, 85.2511) (-197.2897, 85.4533) knots 0 0 0 0 1 1 1 1
  spline S584 degree 3 poles (-197.2897, 85.4533) (-196.8565, 85.9732) (-196.712, 86.1899) (-196.4088, 86.7892) knots 0 0 0 0 1 1 1 1
  spline S585 degree 3 poles (-196.4088, 86.7892) (-196.1271, 87.3524) (-195.8672, 88.2551) (-195.8672, 88.6739) knots 0 0 0 0 1 1 1 1
  spline S586 degree 3 poles (-195.8672, 88.6739) (-195.8672, 88.8761) (-195.8455, 88.9122) (-195.7733, 88.84) knots 0 0 0 0 1 1 1 1
  spline S587 degree 3 poles (-195.7733, 88.84) (-195.7155, 88.775) (-195.6867, 88.5006) (-195.6867, 88.0096) knots 0 0 0 0 1 1 1 1
  spline S588 degree 3 poles (-202.5033, 88.4428) (-202.5755, 88.3778) (-202.5827, 88.3851) (-202.5394, 88.4861) knots 0 0 0 0 1 1 1 1
  spline S589 degree 3 poles (-202.5394, 88.4861) (-202.5178, 88.5584) (-202.4744, 88.5945) (-202.4528, 88.5728) knots 0 0 0 0 1 1 1 1
  spline S590 degree 3 poles (-202.4528, 88.5728) (-202.4311, 88.5511) (-202.4528, 88.4934) (-202.5033, 88.4428) knots 0 0 0 0 1 1 1 1
  spline S591 degree 3 poles (-197.9107, 87.764) (-197.9252, 87.6485) (-197.9396, 87.7279) (-197.9396, 87.9229) knots 0 0 0 0 1 1 1 1
  spline S592 degree 3 poles (-197.9396, 87.9229) (-197.9396, 88.1251) (-197.9252, 88.2117) (-197.9107, 88.1251) knots 0 0 0 0 1 1 1 1
  spline S593 degree 3 poles (-197.9107, 88.1251) (-197.8963, 88.0312) (-197.8963, 87.8724) (-197.9107, 87.764) knots 0 0 0 0 1 1 1 1
  line L96 (-202.3661, 87.533) -> (-201.9762, 87.1864)
  line L97 (-201.9762, 87.1864) -> (-202.3517, 86.3632)
  spline S594 degree 3 poles (-202.3517, 86.3632) (-202.886, 85.1934) (-202.8933, 85.1789) (-203.081, 85.1573) knots 0 0 0 0 1 1 1 1
  spline S595 degree 3 poles (-203.081, 85.1573) (-203.2687, 85.1284) (-203.8103, 85.4605) (-203.8103, 85.5977) knots 0 0 0 0 1 1 1 1
  spline S596 degree 3 poles (-203.8103, 85.5977) (-203.8103, 85.6483) (-203.6442, 86.0815) (-203.442, 86.5509) knots 0 0 0 0 1 1 1 1
  spline S597 degree 3 poles (-203.442, 86.5509) (-203.2399, 87.0275) (-203.0305, 87.5257) (-202.9799, 87.6557) knots 0 0 0 0 1 1 1 1
  spline S598 degree 3 poles (-202.9799, 87.6557) (-202.9221, 87.7785) (-202.8499, 87.8868) (-202.821, 87.8868) knots 0 0 0 0 1 1 1 1
  spline S599 degree 3 poles (-202.821, 87.8868) (-202.7922, 87.8868) (-202.5827, 87.7279) (-202.3661, 87.533) knots 0 0 0 0 1 1 1 1
  spline S600 degree 3 poles (-200.3948, 86.5726) (-200.4092, 86.5365) (-200.3514, 86.5148) (-200.2576, 86.522) knots 0 0 0 0 1 1 1 1
  spline S601 degree 3 poles (-200.2576, 86.522) (-200.1637, 86.522) (-199.8965, 86.4715) (-199.6582, 86.4137) knots 0 0 0 0 1 1 1 1
  spline S602 degree 3 poles (-199.6582, 86.4137) (-199.4199, 86.3487) (-199.0517, 86.2982) (-198.8423, 86.2982) knots 0 0 0 0 1 1 1 1
  spline S603 degree 3 poles (-198.8423, 86.2982) (-198.5029, 86.2982) (-198.4668, 86.2837) (-198.4668, 86.1393) knots 0 0 0 0 1 1 1 1
  spline S604 degree 3 poles (-198.4668, 86.1393) (-198.4668, 85.8721) (-199.16, 85.2728) (-199.7304, 85.0345) knots 0 0 0 0 1 1 1 1
  spline S605 degree 3 poles (-199.7304, 85.0345) (-200.1493, 84.8684) (-200.3731, 84.8251) (-201.0447, 84.7962) knots 0 0 0 0 1 1 1 1
  spline S606 degree 3 poles (-201.0447, 84.7962) (-201.4924, 84.7818) (-201.8606, 84.7745) (-201.8606, 84.789) knots 0 0 0 0 1 1 1 1
  spline S607 degree 3 poles (-201.8606, 84.789) (-201.8606, 84.9406) (-201.2108, 86.3632) (-201.0591, 86.5581) knots 0 0 0 0 1 1 1 1
  spline S608 degree 3 poles (-201.0591, 86.5581) (-200.9869, 86.6448) (-200.337, 86.6592) (-200.3948, 86.5726) knots 0 0 0 0 1 1 1 1
  spline S609 degree 3 poles (-223.8198, 80.4636) (-223.6754, 80.3047) (-223.6537, 80.2253) (-223.6898, 79.9003) knots 0 0 0 0 1 1 1 1
  spline S610 degree 3 poles (-223.6898, 79.9003) (-223.7404, 79.4237) (-223.8776, 79.1566) (-224.3036, 78.7161) knots 0 0 0 0 1 1 1 1
  spline S611 degree 3 poles (-224.3036, 78.7161) (-224.7152, 78.2973) (-225.0835, 78.1673) (-225.4445, 78.3189) knots 0 0 0 0 1 1 1 1
  spline S612 degree 3 poles (-225.4445, 78.3189) (-225.7623, 78.4489) (-225.8634, 78.7955) (-225.7334, 79.2938) knots 0 0 0 0 1 1 1 1
  spline S613 degree 3 poles (-225.7334, 79.2938) (-225.5673, 79.9292) (-225.1268, 80.4347) (-224.5419, 80.6369) knots 0 0 0 0 1 1 1 1
  spline S614 degree 3 poles (-224.5419, 80.6369) (-224.2242, 80.7524) (-224.0437, 80.7091) (-223.8198, 80.4636) knots 0 0 0 0 1 1 1 1
  spline S615 degree 3 poles (-184.3569, 80.2614) (-184.198, 80.1025) (-184.2124, 79.8931) (-184.393, 79.7992) knots 0 0 0 0 1 1 1 1
  spline S616 degree 3 poles (-184.393, 79.7992) (-184.6313, 79.6693) (-184.7468, 79.7631) (-184.7468, 80.0881) knots 0 0 0 0 1 1 1 1
  spline S617 degree 3 poles (-184.7468, 80.0881) (-184.7468, 80.3264) (-184.7251, 80.3769) (-184.6096, 80.3769) knots 0 0 0 0 1 1 1 1
  spline S618 degree 3 poles (-184.6096, 80.3769) (-184.5302, 80.3769) (-184.4146, 80.3264) (-184.3569, 80.2614) knots 0 0 0 0 1 1 1 1
  spline S619 degree 3 poles (-182.5516, 78.4995) (-182.5083, 77.994) (-182.5227, 77.9434) (-182.7971, 77.7557) knots 0 0 0 0 1 1 1 1
  spline S620 degree 3 poles (-182.7971, 77.7557) (-183.0426, 77.5896) (-183.382, 77.604) (-183.6709, 77.799) knots 0 0 0 0 1 1 1 1
  spline S621 degree 3 poles (-183.6709, 77.799) (-183.9092, 77.9579) (-184.1619, 78.3117) (-184.0897, 78.3839) knots 0 0 0 0 1 1 1 1
  spline S622 degree 3 poles (-184.0897, 78.3839) (-184.0752, 78.4056) (-183.9092, 78.3695) (-183.7358, 78.3117) knots 0 0 0 0 1 1 1 1
  spline S623 degree 3 poles (-183.7358, 78.3117) (-183.2015, 78.124) (-182.826, 78.3117) (-182.7466, 78.8027) knots 0 0 0 0 1 1 1 1
  spline S624 degree 3 poles (-182.7466, 78.8027) (-182.6888, 79.1927) (-182.6094, 79.0627) (-182.5516, 78.4995) knots 0 0 0 0 1 1 1 1
  spline S625 degree 3 poles (-192.9282, 78.4489) (-192.1267, 77.9434) (-192.1484, 77.9651) (-192.1267, 77.6907) knots 0 0 0 0 1 1 1 1
  spline S626 degree 3 poles (-192.1267, 77.6907) (-192.105, 77.4668) (-192.1411, 77.4019) (-192.3578, 77.2358) knots 0 0 0 0 1 1 1 1
  spline S627 degree 3 poles (-192.3578, 77.2358) (-192.6538, 77.0119) (-192.6683, 76.9325) (-192.4805, 76.557) knots 0 0 0 0 1 1 1 1
  spline S628 degree 3 poles (-192.4805, 76.557) (-192.2494, 76.1093) (-191.874, 75.8277) (-191.5129, 75.8277) knots 0 0 0 0 1 1 1 1
  spline S629 degree 3 poles (-191.5129, 75.8277) (-191.3468, 75.8277) (-191.1302, 75.8782) (-191.0435, 75.9432) knots 0 0 0 0 1 1 1 1
  spline S630 degree 3 poles (-191.0435, 75.9432) (-190.7908, 76.1165) (-190.5958, 76.5787) (-190.5381, 77.1491) knots 0 0 0 0 1 1 1 1
  line L98 (-190.5381, 77.1491) -> (-190.4875, 77.669)
  line L99 (-190.4875, 77.669) -> (-190.177, 77.734)
  spline S631 degree 3 poles (-190.177, 77.734) (-189.9748, 77.7774) (-189.8376, 77.7701) (-189.7943, 77.7268) knots 0 0 0 0 1 1 1 1
  spline S632 degree 3 poles (-189.7943, 77.7268) (-189.6643, 77.5968) (-189.7004, 76.5353) (-189.8376, 76.1165) knots 0 0 0 0 1 1 1 1
  spline S633 degree 3 poles (-189.8376, 76.1165) (-189.9748, 75.6977) (-190.2925, 75.3005) (-190.6175, 75.1272) knots 0 0 0 0 1 1 1 1
  spline S634 degree 3 poles (-190.6175, 75.1272) (-190.9569, 74.9539) (-191.6573, 74.9756) (-192.0617, 75.1706) knots 0 0 0 0 1 1 1 1
  spline S635 degree 3 poles (-192.0617, 75.1706) (-192.5094, 75.3872) (-192.791, 75.741) (-193.0149, 76.362) knots 0 0 0 0 1 1 1 1
  spline S636 degree 3 poles (-193.0149, 76.362) (-193.3543, 77.308) (-193.5348, 78.6439) (-193.3326, 78.6439) knots 0 0 0 0 1 1 1 1
  spline S637 degree 3 poles (-193.3326, 78.6439) (-193.2893, 78.6439) (-193.1087, 78.5572) (-192.9282, 78.4489) knots 0 0 0 0 1 1 1 1
  spline S638 degree 3 poles (-203.9836, 69.5815) (-203.767, 69.2421) (-204.027, 68.5055) (-204.5108, 68.1084) knots 0 0 0 0 1 1 1 1
  spline S639 degree 3 poles (-204.5108, 68.1084) (-204.814, 67.8557) (-205.0018, 67.8268) (-205.1968, 68.0073) knots 0 0 0 0 1 1 1 1
  spline S640 degree 3 poles (-205.1968, 68.0073) (-205.4784, 68.26) (-205.2979, 69.0038) (-204.8429, 69.4587) knots 0 0 0 0 1 1 1 1
  spline S641 degree 3 poles (-204.8429, 69.4587) (-204.4747, 69.827) (-204.1714, 69.8703) (-203.9836, 69.5815) knots 0 0 0 0 1 1 1 1
  spline S642 degree 3 poles (-179.6343, 69.5815) (-179.3455, 69.3432) (-179.0999, 68.7511) (-179.1288, 68.3683) knots 0 0 0 0 1 1 1 1
  spline S643 degree 3 poles (-179.1288, 68.3683) (-179.1505, 68.0723) (-179.1577, 68.0651) (-179.4754, 68.0073) knots 0 0 0 0 1 1 1 1
  spline S644 degree 3 poles (-179.4754, 68.0073) (-179.6776, 67.9712) (-179.9087, 67.9784) (-180.0748, 68.029) knots 0 0 0 0 1 1 1 1
  spline S645 degree 3 poles (-180.0748, 68.029) (-180.6597, 68.195) (-181.1652, 68.9171) (-180.9991, 69.3504) knots 0 0 0 0 1 1 1 1
  spline S646 degree 3 poles (-180.9991, 69.3504) (-180.8402, 69.762) (-180.017, 69.9064) (-179.6343, 69.5815) knots 0 0 0 0 1 1 1 1
  spline S647 degree 3 poles (-199.2972, 106.0621) (-199.7016, 105.9249) (-199.8821, 105.8239) (-200.2142, 105.5206) knots 0 0 0 0 1 1 1 1
  spline S648 degree 3 poles (-200.2142, 105.5206) (-200.5464, 105.2245) (-200.6692, 105.0007) (-200.7775, 104.5313) knots 0 0 0 0 1 1 1 1
  spline S649 degree 3 poles (-200.7775, 104.5313) (-200.8641, 104.1558) (-200.7703, 103.4626) (-200.597, 103.1232) knots 0 0 0 0 1 1 1 1
  spline S650 degree 3 poles (-200.597, 103.1232) (-200.0482, 102.0617) (-198.0913, 101.614) (-197.2031, 102.3433) knots 0 0 0 0 1 1 1 1
  spline S651 degree 3 poles (-197.2031, 102.3433) (-196.7987, 102.6827) (-196.6615, 103.0365) (-196.6615, 103.7875) knots 0 0 0 0 1 1 1 1
  spline S652 degree 3 poles (-196.6615, 103.7875) (-196.6615, 104.8707) (-197.037, 105.5495) (-197.853, 105.9322) knots 0 0 0 0 1 1 1 1
  spline S653 degree 3 poles (-197.853, 105.9322) (-198.2862, 106.1344) (-198.9, 106.1921) (-199.2972, 106.0621) knots 0 0 0 0 1 1 1 1
  spline S654 degree 3 poles (-198.084, 104.423) (-197.7663, 104.0619) (-197.8602, 103.6214) (-198.3007, 103.4409) knots 0 0 0 0 1 1 1 1
  spline S655 degree 3 poles (-198.3007, 103.4409) (-198.8278, 103.2171) (-199.3333, 103.5492) (-199.3333, 104.1197) knots 0 0 0 0 1 1 1 1
  spline S656 degree 3 poles (-199.3333, 104.1197) (-199.3333, 104.7046) (-198.5173, 104.9068) (-198.084, 104.423) knots 0 0 0 0 1 1 1 1
  spline S657 degree 3 poles (-213.0605, 72.636) (-213.1688, 72.506) (-213.5876, 71.9789) (-213.992, 71.4662) knots 0 0 0 0 1 1 1 1
  spline S658 degree 3 poles (-213.992, 71.4662) (-214.3964, 70.9607) (-214.9018, 70.3469) (-215.1185, 70.1158) knots 0 0 0 0 1 1 1 1
  spline S659 degree 3 poles (-215.1185, 70.1158) (-215.3351, 69.8848) (-215.5084, 69.6465) (-215.5084, 69.5887) knots 0 0 0 0 1 1 1 1
  spline S660 degree 3 poles (-215.5084, 69.5887) (-215.5084, 69.5237) (-215.3784, 69.4804) (-215.1112, 69.4515) knots 0 0 0 0 1 1 1 1
  spline S661 degree 3 poles (-215.1112, 69.4515) (-213.8909, 69.3287) (-213.0099, 68.3756) (-212.5911, 66.7292) knots 0 0 0 0 1 1 1 1
  spline S662 degree 3 poles (-212.5911, 66.7292) (-212.5044, 66.3753) (-212.4106, 66.0576) (-212.3817, 66.036) knots 0 0 0 0 1 1 1 1
  spline S663 degree 3 poles (-212.3817, 66.036) (-212.36, 66.0143) (-212.1217, 66.0937) (-211.8618, 66.2165) knots 0 0 0 0 1 1 1 1
  spline S664 degree 3 poles (-211.8618, 66.2165) (-211.5224, 66.3826) (-211.1469, 66.4837) (-210.6053, 66.5559) knots 0 0 0 0 1 1 1 1
  spline S665 degree 3 poles (-210.6053, 66.5559) (-210.1865, 66.6209) (-209.7749, 66.7147) (-209.6955, 66.7653) knots 0 0 0 0 1 1 1 1
  spline S666 degree 3 poles (-209.6955, 66.7653) (-209.6088, 66.8158) (-209.4066, 67.2202) (-209.1972, 67.7473) knots 0 0 0 0 1 1 1 1
  spline S667 degree 3 poles (-209.1972, 67.7473) (-209.0022, 68.2384) (-208.6701, 69.011) (-208.4607, 69.4659) knots 0 0 0 0 1 1 1 1
  spline S668 degree 3 poles (-208.4607, 69.4659) (-208.244, 69.9209) (-208.0707, 70.3397) (-208.0707, 70.4119) knots 0 0 0 0 1 1 1 1
  spline S669 degree 3 poles (-208.0707, 70.4119) (-208.0707, 70.4913) (-208.7278, 70.8524) (-210.3237, 71.6539) knots 0 0 0 0 1 1 1 1
  spline S670 degree 3 poles (-210.3237, 71.6539) (-211.5657, 72.2749) (-212.6416, 72.8021) (-212.7211, 72.8237) knots 0 0 0 0 1 1 1 1
  spline S671 degree 3 poles (-212.7211, 72.8237) (-212.815, 72.8598) (-212.916, 72.8021) (-213.0605, 72.636) knots 0 0 0 0 1 1 1 1
  spline S672 degree 3 poles (-209.3922, 69.9209) (-209.4138, 69.8559) (-209.6088, 69.3793) (-209.8327, 68.8594) knots 0 0 0 0 1 1 1 1
  spline S673 degree 3 poles (-209.8327, 68.8594) (-210.0565, 68.3467) (-210.2659, 67.8557) (-210.302, 67.7762) knots 0 0 0 0 1 1 1 1
  spline S674 degree 3 poles (-210.302, 67.7762) (-210.3526, 67.6535) (-210.4753, 67.6101) (-210.9375, 67.5451) knots 0 0 0 0 1 1 1 1
  spline S675 degree 3 poles (-210.9375, 67.5451) (-211.248, 67.5018) (-211.5441, 67.4513) (-211.5946, 67.4368) knots 0 0 0 0 1 1 1 1
  spline S676 degree 3 poles (-211.5946, 67.4368) (-211.6451, 67.4224) (-211.7896, 67.6535) (-211.9195, 67.9567) knots 0 0 0 0 1 1 1 1
  spline S677 degree 3 poles (-211.9195, 67.9567) (-212.3167, 68.8594) (-212.815, 69.4876) (-213.4721, 69.9064) knots 0 0 0 0 1 1 1 1
  line L100 (-213.4721, 69.9064) -> (-213.7754, 70.1086)
  line L101 (-213.7754, 70.1086) -> (-213.1616, 70.874)
  line L102 (-213.1616, 70.874) -> (-212.5478, 71.6395)
  line L103 (-212.5478, 71.6395) -> (-210.9519, 70.8379)
  spline S678 degree 3 poles (-210.9519, 70.8379) (-209.6738, 70.2025) (-209.3633, 70.022) (-209.3922, 69.9209) knots 0 0 0 0 1 1 1 1